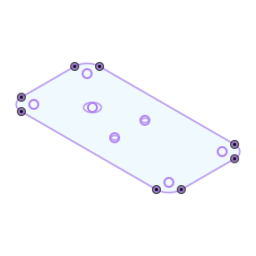
uchwyt do silika v2 (Autodesk Fusion 360 design; units mm, degrees)
Autodesk Fusion 360 part; units mm, degrees
sketch "Sketch1" plane through (0, 0, 0) normal (0, 1, 0) x (1, 0, 0)
  line L0 (7, 0) -> (83, 0)
  line L1 (90, 7) -> (90, 37)
  line L2 (83, 44) -> (7, 44)
  line L3 (0, 37) -> (0, 7)
  line L4 (0, 22) -> (90, 22) construction
  circle A0 centre (25, 22) radius 3.5
  circle A1 centre (25, 22) radius 32.5 construction
  arc A2 (7, 44) -> (0, 37) centre (7, 37) ccw
  arc A3 (90, 37) -> (83, 44) centre (83, 37) ccw
  arc A4 (0, 7) -> (7, 0) centre (7, 7) ccw
  arc A5 (83, 0) -> (90, 7) centre (83, 7) ccw
  line L5 (46, 63.3038) -> (46, -13) construction
  circle A6 centre (46, 30.5) radius 1.5
  circle A7 centre (46, 13.5) radius 1.5
  point P0 (90, 0)
  point P1 (0, 44)
  dimension "szerokosc" = 90
  dimension "wysokosc" = 44
  dimension "d_osi" = 7
  dimension "d4" = 25
  dimension "d_kola" = 65
  dimension "d6" = 7
  dimension "d7" = 7
  dimension "d8" = 7
  dimension "d9" = 7
  dimension "d10" = 3
  dimension "d11" = 3
  dimension "miedzy_otworami" = 17
  dimension "d13" = 8.5
  dimension "d14" = 21
  constraint horizontal L0
  constraint vertical L1
  constraint horizontal L2
  constraint vertical L3
  constraint coincident L4 A0.centre
  constraint concentric A0 A1
  constraint coincident L3 L4.start
  constraint coincident P1 L2
  constraint coincident P1 L3
  constraint tangent L2 A2
  constraint tangent L3 A2
  constraint coincident L1 L4.end
  constraint tangent L1 A3
  constraint tangent L2 A3
  constraint coincident origin L0
  constraint coincident origin L3
  constraint tangent L0 A4
  constraint tangent L3 A4
  constraint coincident P0 L0
  constraint coincident P0 L1
  constraint tangent L0 A5
  constraint tangent L1 A5
  constraint perpendicular L4 L5
  constraint coincident L5 A6.centre
  constraint coincident L5 A7.centre
  constraint vertical L5
  measures "szerokosc" distance of origin P0
  measures "wysokosc" distance of origin P1
  measures "d_osi" diameter of A0
  measures "d4" distance of L3 A0.centre
  measures "d_kola" diameter of A1
  measures "d6" radius of A2
  measures "d7" radius of A3
  measures "d8" radius of A4
  measures "d9" radius of A5
  measures "d10" diameter of A6
  measures "d11" diameter of A7
  measures "miedzy_otworami" distance of A6.centre A7.centre
  measures "d13" distance of L4 A6.centre
  measures "d14" distance of A0.centre L5
extrude "Extrude1" add sketch "Sketch1" along normal blind 3
sketch "Sketch2" plane through (0, 3, 0) normal (0, 1, 0) x (-1, 0, 0)
  circle A0 centre (-25, -22) radius 3.5
  circle A1 centre (-46, -30.5) radius 1.5
  circle A2 centre (-46, -13.5) radius 1.5
  arc A3 (-83, 0) -> (-90, -7) centre (-83, -7) ccw
  line L0 (-90, -7) -> (-90, -37)
  arc A4 (-90, -37) -> (-83, -44) centre (-83, -37) ccw
  line L1 (-83, -44) -> (-7, -44)
  arc A5 (-7, -44) -> (0, -37) centre (-7, -37) ccw
  line L2 (0, -37) -> (0, -7)
  arc A6 (0, -7) -> (-7, 0) centre (-7, -7) ccw
  line L3 (-7, 0) -> (-83, 0)
equation "wysokosc = szerokosc / 3 + 2 * d_osi"
equation "d6 = d_osi"
equation "d7 = d_osi"
equation "d8 = d_osi"
equation "d9 = d_osi"
equation "miedzy_otworami = 20 mm - 3 mm"
equation "d13 = miedzy_otworami / 2"
